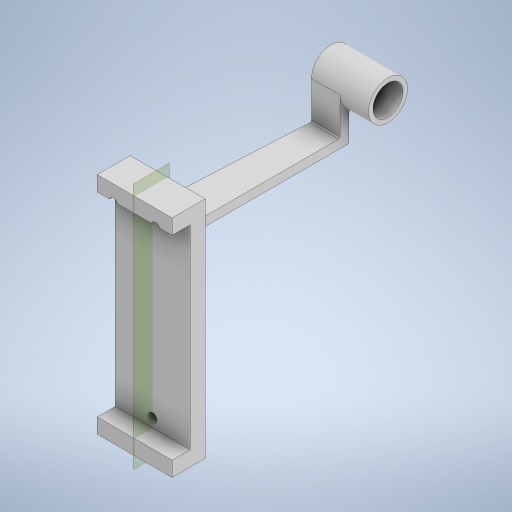
# Autodesk Inventor part: 6 - Part 6
Saved by Autodesk Inventor 2024 (Build 280153000, 153)
## iProperties
Created: 2024-04-21
Part Number: 6 - Part 6
Material: Generic
Document SubType Name: Modeling
Designer: Ricsi
Density: 1 g/cm^3
Appearance: Default
Author: Ricsi
Autodesk Inventor part; units mm, degrees
ref_plane "YZ Plane" through (0, 0, 0) normal (1, 0, 0) x (0, 1, 0)
ref_plane "XZ Plane" through (0, 0, 0) normal (0, 1, 0) x (-1, 0, 0)
ref_plane "XY Plane" through (0, 0, 0) normal (0, 0, 1) x (1, 0, 0)
sketch "Sketch1" plane through (0, 0, 0) normal (0, 0, 1) x (1, 0, 0)
  line L0 (-113.263, 0) -> (-213.263, 0)
  line L1 (-213.263, 0) -> (-213.263, 300)
  line L2 (-213.263, 300) -> (-113.263, 300)
  line L3 (-113.263, 300) -> (-113.263, 0)
  circle A0 centre (-163.263, 32) radius 6
  circle A1 centre (-191.263, 278) radius 6
  circle A2 centre (-135.263, 278) radius 6
  point P0 (0, 0)
  dimension "d0" = 100
  dimension "d1" = 300
  dimension "d2" = 12
  dimension "d3" = 32
  dimension "d4" = 12
  dimension "d5" = 22
  dimension "d6" = 22
  dimension "d7" = 12
  dimension "d8" = 22
  dimension "d9" = 22
  constraints: 8 end point, 3 centre point, 2 parallel, 1 horizontal, 1 perpendicular
  measures "d0" distance of L1.end L2.end
  measures "d1" distance of L0.end L1.end
  measures "d2" diameter of A0
  measures "d3" distance from line of L0 A0.centre
  measures "d4" diameter of A1
  measures "d5" distance from line of L2 A1.centre
  measures "d6" distance from line of L1 A1.centre
  measures "d7" diameter of A2
  measures "d8" distance from line of L2 A2.centre
  measures "d9" distance from line of L3 A2.centre
extrude "Extrusion1" add sketch "Sketch1" along normal blind 44
sketch "Sketch2" plane through (0, 0, 44) normal (0, 0, 1) x (1, 0, 0)
  line L0 (-113.263, 300) -> (-213.263, 300) projected
  line L1 (-213.263, 300) -> (-213.263, 280)
  line L2 (-213.263, 300) -> (-213.263, 0) projected
  line L3 (-213.263, 280) -> (-113.263, 280)
  line L4 (-113.263, 0) -> (-113.263, 300) projected
  line L5 (-113.263, 280) -> (-113.263, 300)
  line L6 (-213.263, 300) -> (-113.263, 300)
  line L7 (-213.263, 0) -> (-213.263, 20)
  line L8 (-213.263, 0) -> (-113.263, 0) projected
  line L9 (-213.263, 0) -> (-113.263, 0)
  line L10 (-113.263, 0) -> (-113.263, 20)
  line L11 (-213.263, 20) -> (-113.263, 20)
  line L12 (-113.263, 20) -> (-113.263, 280)
  line L13 (-213.263, 20) -> (-213.263, 280)
  point P0 (0, 0)
  dimension "d12" = 20
  dimension "d13" = 20
  constraints: 20 end point, 4 collinear, 4 point on line, 2 perpendicular, 1 horizontal
  measures "d12" distance of L0.end L1.end
  measures "d13" distance of L2.end L7.end
extrude "Extrusion2" cut sketch "Sketch2" against normal blind 24 contours L4 L11 L2 L3
ref_plane "Work Plane1" through (-163.263, 0, 0) normal (-1, 0, 0) x (0, 0, 1)
sketch "Sketch6" plane through (-163.263, 0, 0) normal (-1, 0, 0) x (0, 0, 1)
  line L0 (44, 284) -> (44, 280) projected
  circle A0 centre (-256, 280) radius 26
  point P0 (0, 0)
  dimension "d24" = 52
  constraints: 1 centre point
  measures "d24" diameter of A0
extrude "Extrusion5" add sketch "Sketch6" along normal mid plane 76
sketch "Sketch7" plane through (-201.263, 280, -256) normal (-1, 0, 0) x (0, 0, 1)
  circle A0 centre (0, 0) radius 20
  point P0 (256, -280)
  dimension "d27" = 40
  constraints: 1 centre point
  measures "d27" diameter of A0
extrude "Extrusion6" cut sketch "Sketch7" against normal blind 76
sketch "Sketch9" plane through (-163.263, 0, 0) normal (-1, 0, 0) x (0, 0, 1)
  line L0 (44, 284) -> (44, 280) projected
  circle A0 centre (-256, 280) radius 26
  line L1 (0, 300) -> (0, 0) projected
  circle A1 centre (-256, 280) radius 26 projected
  line L2 (0, 230) -> (-228, 230)
  line L3 (-230, 232) -> (-230, 280)
  line L4 (0, 230) -> (0, 218)
  line L5 (0, 218) -> (-240, 218)
  line L6 (-242, 220) -> (-242, 253)
  arc A2 (-230, 232) -> (-228, 230) centre (-228, 232) ccw
  arc A3 (-242, 220) -> (-240, 218) centre (-240, 220) ccw
  line L7 (-242, 253) -> (-250.7822, 253) construction
  line L8 (-243.1836, 257.3871) -> (-250.7822, 253) construction
  arc A4 (-242, 253) -> (-243.1836, 257.3871) centre (-250.7225, 253) ccw
  point P0 (-242, 218)
  point P1 (-243.1797, 257.3805)
  dimension "d35" = 52
  dimension "d37" = 12
  dimension "d38" = 242
  dimension "d39" = 35
  dimension "d40" = 2
  dimension "d41" = 2
  dimension "d42" = 30
  constraints: 14 end point, 6 point on circle, 5 tangent, 4 centre point, 4 point on line, 2 vertical, 1 horizontal alignment, 1 perpendicular, 1 other
  measures "d35" diameter of A0
  measures "d37" distance of L2.start L4.end
  measures "d38" distance of L4.end point (-242, 218)
  measures "d39" distance of point (-242, 218) L6.end
  measures "d40" radius of A2
  measures "d41" radius of A3
  measures "d42" angle of L7 L8
extrude "Extrusion7" add sketch "Sketch9" along normal blind 50 contours L3 A2 L2 L1 L5 A3 L6 A4 A0
sketch "Sketch10" plane through (-163.263, 230, 0) normal (0, 1, 0) x (1, 0, 0)
  line L0 (-50, 0) -> (-41.2717, 264.4302)
  line L1 (-41.2717, 264.4302) -> (-54.1734, 264.856)
  line L2 (-54.1734, 264.856) -> (-50, 0)
  point P0 (163.263, 0)
  constraints: 6 end point, 1 perpendicular
extrude "Extrusion8" cut sketch "Sketch10" against normal blind 50
sketch "Sketch12" plane through (-213.263, 232, -230) normal (-1, 0, 0) x (0, 0, 1)
  line L0 (-12, 21) -> (-12, -2) projected
  line L1 (0, 48) -> (2.6747, 48)
  line L2 (-12, 48) -> (0, 48)
  line L3 (2.6747, 48) -> (2.6747, -2)
  line L4 (2, -2) -> (230, -2) projected
  line L5 (-12, -2) -> (2.6747, -2)
  line L6 (-12, -2) -> (-15.3342, -2)
  line L7 (-15.3342, -2) -> (-15.3342, 48)
  line L8 (-15.3342, 48) -> (-11.4757, 48)
  point P0 (230, -232)
  constraints: 14 end point, 3 point on line, 2 horizontal, 2 perpendicular, 1 collinear
extrude "Extrusion9" cut sketch "Sketch12" against normal blind 12
sketch "Sketch13" plane through (-163.263, 230, 0) normal (0, 1, 0) x (1, 0, 0)
  line L0 (-38, 228) -> (-38, 242) projected
  line L1 (-38, 228) -> (-50, 0)
  line L2 (-42.012, 242) -> (-38, 242) projected
  line L3 (-50, 0) -> (-42.012, 242)
  line L4 (-42.012, 242) -> (-38, 242)
  line L5 (-38, 242) -> (-38, 228)
  point P0 (163.263, 0)
  constraints: 8 end point, 1 collinear, 1 perpendicular
extrude "Extrusion10" cut sketch "Sketch13" against normal blind 12
body "Solid1"
